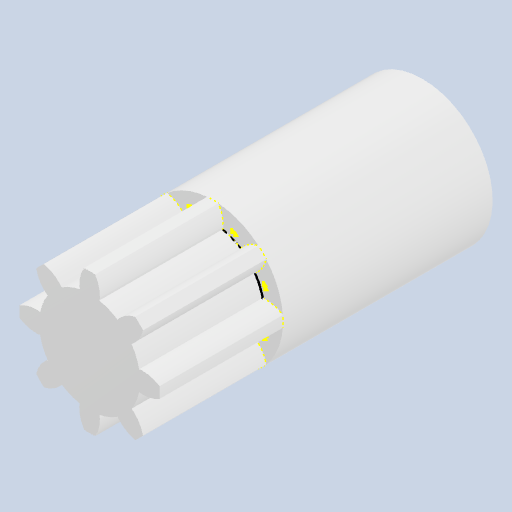
# Autodesk Inventor part: Pinion_V2
Saved by Autodesk Inventor 2024 (Build 280153000, 153)
## iProperties
Created: 2023-12-09
Part Number: Pinion_V2
Material: Polystyrene
Document SubType Name: Modeling
Designer: mirun
Density: 1.021 g/cm^3
Appearance: Smooth - White
Author: mirun
Autodesk Inventor part; units mm, degrees
ref_plane "YZ Plane" through (0, 0, 0) normal (1, 0, 0) x (0, 1, 0)
ref_plane "XZ Plane" through (0, 0, 0) normal (0, 1, 0) x (-1, 0, 0)
ref_plane "XY Plane" through (0, 0, 0) normal (0, 0, 1) x (1, 0, 0)
sketch "Sketch1" plane through (0, 0, 0) normal (0, 0, 1) x (1, 0, 0)
  arc A0 (0, 5) -> (0.7683, 4.9406) centre (0, 0) ccw construction
  arc A1 (0, 5.7) -> (0.45, 5.6822) centre (0, 0) ccw
  arc A2 (0, 4.3) -> (0.839, 4.2174) centre (0, 0) ccw construction
  arc A3 (0, 4.1002) -> (0.8, 4.0214) centre (0, 0) ccw
  arc A4 (-0.45, 5.6822) -> (-0.839, 4.2174) centre (1.6581, 4.3383) ccw
  line L0 (-0.839, 4.2174) -> (-0.8, 4.0214)
  line L1 (0, 0) -> (0, 10.8363)
  arc A5 (0.839, 4.2174) -> (0.45, 5.6822) centre (-1.6581, 4.3383) ccw
  line L2 (0.839, 4.2174) -> (0.8, 4.0214)
  arc A6 (0.45, 5.6822) -> (0, 5.7) centre (0, 0) ccw
  arc A7 (0.7683, 4.9406) -> (0, 5) centre (0, 0) ccw construction
  arc A8 (0.839, 4.2174) -> (0, 4.3) centre (0, 0) ccw construction
  arc A9 (0.8, 4.0214) -> (0, 4.1002) centre (0, 0) ccw
  circle A10 centre (0, 0) radius 3.25
  point P0 (0.455, 5.6318)
  point P1 (0.3281, 6.8421)
  dimension "d0" = 10
  dimension "d8" = 2.5
  dimension "d14" = 0.7
  dimension "d15" = 0.7
  dimension "d16" = 0.1998
  dimension "d17" = 0.8
  dimension "d18" = 0.45
  dimension "d19" = 6.5
  constraints: 24 point on circle, 11 centre point, 6 end point, 5 coincident, 4 point on line, 4 symmetric about line, 1 line through centre, 1 vertical, 1 other
  measures "d0" diameter of A0
  measures "d8" radius of A4
  measures "d14" distance of A0.start A1.start
  measures "d15" distance of A2.start A0.start
  measures "d16" distance of A3.start A2.start
  measures "d17" horizontal distance of L0.end A3.start
  measures "d18" horizontal distance of A4.start A1.start
  measures "d19" diameter of A10
extrude "Extrusion1" add sketch "Sketch1" along normal blind 10 contours L1 A3 L0 A4 A1 | A6 A5 L2 A9 L1 | A9 A3 | A10
pattern_circular "Circular Pattern1" count 8 over 360 about axis through (0, 0, 0) along (0, 0, 1) of "Extrusion1"
sketch "Sketch2" plane through (0, 0, 0) normal (0, 0, -1) x (-1, 0, 0)
  line L0 (0.839, 4.2174) -> (0.8, 4.0214) construction
  arc A0 (0.839, 4.2174) -> (0.45, 5.6822) centre (-1.6581, 4.3383) ccw construction
  arc A1 (0.45, 5.6822) -> (-0.45, 5.6822) centre (0, 0) ccw construction
  arc A2 (-0.45, 5.6822) -> (-0.839, 4.2174) centre (1.6581, 4.3383) ccw construction
  line L1 (-0.8, 4.0214) -> (-0.839, 4.2174) construction
  arc A3 (-0.8, 4.0214) -> (-2.2779, 3.4092) centre (0, 0) ccw construction
  line L2 (-2.3889, 3.5754) -> (-2.2779, 3.4092) construction
  arc A4 (-2.3889, 3.5754) -> (-3.6997, 4.3361) centre (-4.2401, 1.8952) ccw construction
  arc A5 (-3.6997, 4.3361) -> (-4.3361, 3.6997) centre (0, 0) ccw construction
  arc A6 (-4.3361, 3.6997) -> (-3.5754, 2.3889) centre (-1.8952, 4.2401) ccw construction
  line L3 (-3.4092, 2.2779) -> (-3.5754, 2.3889) construction
  arc A7 (-3.4092, 2.2779) -> (-4.0214, 0.8) centre (0, 0) ccw construction
  line L4 (-4.2174, 0.839) -> (-4.0214, 0.8) construction
  arc A8 (-4.2174, 0.839) -> (-5.6822, 0.45) centre (-4.3383, -1.6581) ccw construction
  arc A9 (-5.6822, 0.45) -> (-5.6822, -0.45) centre (0, 0) ccw construction
  arc A10 (-5.6822, -0.45) -> (-4.2174, -0.839) centre (-4.3383, 1.6581) ccw construction
  line L5 (-4.0214, -0.8) -> (-4.2174, -0.839) construction
  arc A11 (-4.0214, -0.8) -> (-3.4092, -2.2779) centre (0, 0) ccw construction
  line L6 (-3.5754, -2.3889) -> (-3.4092, -2.2779) construction
  arc A12 (-3.5754, -2.3889) -> (-4.3361, -3.6997) centre (-1.8952, -4.2401) ccw construction
  arc A13 (-4.3361, -3.6997) -> (-3.6997, -4.3361) centre (0, 0) ccw construction
  arc A14 (-3.6997, -4.3361) -> (-2.3889, -3.5754) centre (-4.2401, -1.8952) ccw construction
  line L7 (-2.2779, -3.4092) -> (-2.3889, -3.5754) construction
  arc A15 (-2.2779, -3.4092) -> (-0.8, -4.0214) centre (0, 0) ccw construction
  line L8 (-0.839, -4.2174) -> (-0.8, -4.0214) construction
  arc A16 (-0.839, -4.2174) -> (-0.45, -5.6822) centre (1.6581, -4.3383) ccw construction
  arc A17 (-0.45, -5.6822) -> (0.45, -5.6822) centre (0, 0) ccw construction
  arc A18 (0.45, -5.6822) -> (0.839, -4.2174) centre (-1.6581, -4.3383) ccw construction
  line L9 (0.8, -4.0214) -> (0.839, -4.2174) construction
  arc A19 (0.8, -4.0214) -> (2.2779, -3.4092) centre (0, 0) ccw construction
  line L10 (2.3889, -3.5754) -> (2.2779, -3.4092) construction
  arc A20 (2.3889, -3.5754) -> (3.6997, -4.3361) centre (4.2401, -1.8952) ccw construction
  arc A21 (3.6997, -4.3361) -> (4.3361, -3.6997) centre (0, 0) ccw construction
  arc A22 (4.3361, -3.6997) -> (3.5754, -2.3889) centre (1.8952, -4.2401) ccw construction
  line L11 (3.4092, -2.2779) -> (3.5754, -2.3889) construction
  arc A23 (3.4092, -2.2779) -> (4.0214, -0.8) centre (0, 0) ccw construction
  line L12 (4.2174, -0.839) -> (4.0214, -0.8) construction
  arc A24 (4.2174, -0.839) -> (5.6822, -0.45) centre (4.3383, 1.6581) ccw construction
  arc A25 (5.6822, -0.45) -> (5.6822, 0.45) centre (0, 0) ccw construction
  arc A26 (5.6822, 0.45) -> (4.2174, 0.839) centre (4.3383, -1.6581) ccw construction
  line L13 (4.0214, 0.8) -> (4.2174, 0.839) construction
  arc A27 (4.0214, 0.8) -> (3.4092, 2.2779) centre (0, 0) ccw construction
  line L14 (3.5754, 2.3889) -> (3.4092, 2.2779) construction
  arc A28 (3.5754, 2.3889) -> (4.3361, 3.6997) centre (1.8952, 4.2401) ccw construction
  arc A29 (4.3361, 3.6997) -> (3.6997, 4.3361) centre (0, 0) ccw construction
  arc A30 (3.6997, 4.3361) -> (2.3889, 3.5754) centre (4.2401, 1.8952) ccw construction
  line L15 (2.2779, 3.4092) -> (2.3889, 3.5754) construction
  arc A31 (2.2779, 3.4092) -> (0.8, 4.0214) centre (0, 0) ccw construction
  circle A32 centre (0, 0) radius 4.1002
  constraints: 1 centre point, 1 coincident, 1 concentric
extrude "Extrusion2" add sketch "Sketch1" against normal blind 17 contours L1 A3 L0 A4 A1 | A6 A5 L2 A9 L1 | A4 L0 A3 L2 A5 A1 | A9 A3 | A10
sketch "Sketch3" plane through (0, 0, -17) normal (0, 0, -1) x (-1, 0, 0)
  circle A0 centre (0, 0) radius 3.25 construction
  circle A1 centre (0, 0) radius 4
  line L0 (-3.5, -1.9365) -> (-3.5, 1.9365)
  line L1 (0, 0) -> (0, 1.4269) construction
  line L2 (3.5, -1.9365) -> (3.5, 1.9365)
  dimension "d22" = 8
  dimension "d23" = 3.5
  constraints: 6 end point, 2 point on circle, 2 symmetric about line, 2 vertical, 1 centre point, 1 coincident
  measures "d22" diameter of A1
  measures "d23" distance between parallel lines of L1 L0
extrude "Extrusion3" cut sketch "Sketch3" against normal blind 15 contours L2 A1 L0
sketch "Sketch4" plane through (0, 0, -17) normal (0, 0, -1) x (-1, 0, 0)
  circle A0 centre (0, 0) radius 5.7 construction
  circle A1 centre (0, 0) radius 4
  point P0 (-3.5, -1.9365)
  constraints: 1 coincident, 3 other
extrude "Extrusion4" cut sketch "Sketch4" against normal blind 2.5
body "Solid1"
